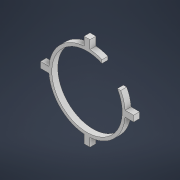
# Autodesk Inventor part: Clip_TestFitV1
Saved by Autodesk Inventor 2022 (Build 260153000, 153)
## iProperties
Created: 2023-05-05
Part Number: Clip_TestFitV1
Material: Generic
Document SubType Name: Modeling
Designer: User
Density: 1 g/cm^3
Appearance: Default
Author: User
Autodesk Inventor part; units mm, degrees
ref_plane "YZ Plane" through (0, 0, 0) normal (1, 0, 0) x (0, 1, 0)
ref_plane "XZ Plane" through (0, 0, 0) normal (0, 1, 0) x (-1, 0, 0)
ref_plane "XY Plane" through (0, 0, 0) normal (0, 0, 1) x (1, 0, 0)
sketch "Sketch1" plane through (0, 0, 0) normal (0, 0, 1) x (1, 0, 0)
  arc A0 (-25.4018, 15) -> (25.4018, 15) centre (0, 0) ccw
  line L0 (25.4018, 15) -> (28.2666, 15)
  line L1 (-39, 2.5) -> (-32, 2.5)
  line L2 (-32, -2.5) -> (-39, -2.5)
  line L3 (-39, -2.5) -> (-39, 2.5)
  line L4 (-32, 2.5) -> (-31.9022, 2.5)
  line L5 (-32, -2.5) -> (-31.9022, -2.5)
  line L6 (2.5, -32) -> (2.5, -39)
  line L7 (2.5, -39) -> (-2.5, -39)
  line L8 (-2.5, -39) -> (-2.5, -32)
  line L9 (-2.5, -32) -> (-2.5, -31.9022)
  line L10 (2.5, -32) -> (2.5, -31.9022)
  line L11 (32, 2.5) -> (39, 2.5)
  line L12 (39, 2.5) -> (39, -2.5)
  line L13 (39, -2.5) -> (32, -2.5)
  line L14 (32, 2.5) -> (31.9022, 2.5)
  line L15 (32, -2.5) -> (31.9022, -2.5)
  arc A1 (-28.2666, 15) -> (-31.9022, 2.5) centre (0, 0) ccw
  arc A2 (-31.9022, -2.5) -> (-2.5, -31.9022) centre (0, 0) ccw
  arc A3 (2.5, -31.9022) -> (31.9022, -2.5) centre (0, 0) ccw
  arc A4 (31.9022, 2.5) -> (28.2666, 15) centre (0, 0) ccw
  arc A5 (12.5, 26.7208) -> (25.4018, 15) centre (0, 0) ccw
  line L16 (-2.5, 31.9022) -> (-2.5, 39.0002)
  line L17 (-2.5, 39.0002) -> (2.5, 39.0002)
  line L18 (2.5, 39.0002) -> (2.5, 31.9022)
  line L19 (12.5, 29.4576) -> (12.5, 26.7208)
  arc A6 (12.5, 29.4576) -> (2.5, 31.9022) centre (0, 0) ccw
  arc A7 (-2.5, 31.9022) -> (-31.9022, 2.5) centre (0, 0) ccw
  arc A8 (-31.9022, -2.5) -> (-2.5, -31.9022) centre (0, 0) ccw
  arc A9 (2.5, -31.9022) -> (31.9022, -2.5) centre (0, 0) ccw
  arc A10 (31.9022, 2.5) -> (28.2666, 15) centre (0, 0) ccw
  constraints: 40 end point, 22 point on circle, 11 centre point, 6 horizontal, 4 parallel, 3 coincident, 2 vertical, 1 perpendicular
extrude "Extrusion5" add sketch "Sketch1" along normal blind 5
body "Solid3"
